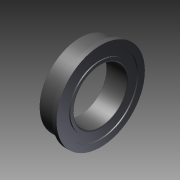
# Autodesk Inventor part: FL6700ZZ
Saved by Autodesk Inventor 2011 SP1 (Build 150282100, 282)
## iProperties
Created: 2017-08-07
Part Number: FL6700ZZ
Catalog Web Link: www.cadenas.de
Description: FL6 _ _ ZZ, FL6 _ _ AZZ, SFL6 _ _ ZZ, SFL6 _ _ AZZ, MFL1 _ _ ZZ, SMFL1 _ _ ZZ-Flanged Ball Bearings (Small Diameter, Deep Groove) - Double Shield Type
Vendor: MISUMI
Document SubType Name: Modeling
Designer: psAdmin
Manufacturer: MISUMI
Mass: 0.398617 g
Surface Area: 6.32309 cm^2
Volume: 0.398617 cm^3
Density: 1 g/cm^3
Category: PARTsolutions
Company: MISUMI
Title: FL6700ZZ
Author: Cadenas PARTsolutions
Comments: Flanged Ball Bearings (Small Diameter, Deep Groove) - Double Shield Type
PSOL_IDENT_0: {$CADENAS_DATA\23d-libs\misumi\metric\12_bearing_holders\sfl608zz.prj},233 {VTYP=3D},{NB=FL6700ZZ},{
PSOL_IDENT_1: LINA=FL6700ZZ},{NN=FL6 _ _ ZZ, FL6 _ _ AZZ, SFL6 _ _ ZZ, SFL6 _ _ AZZ, MFL1 _ _ ZZ, SMFL1 _ _ ZZ},{D
PSOL_IDENT_2: ATE=25.04.2017 02:57:50},{GEOMDATE=28.10.2009 00:00:00},{VERSION=},{LINEID=160},{LINESUBID=-1},{WBVA
PSOL_IDENT_3: R=MAT}  {NB=FL6700ZZ},{LINA=FL6700ZZ},{KT=DUMMY},{PN=FL6700ZZ},{MAT=},{MAT1= '', '52100 Bearing Stee
PSOL_IDENT_4: l', 'S', '440C Stainless Steel'},{BN=6700ZZ},{DD=10.0},{AA=3.6000},{BB=0.5000},{C1=0.7000},{D=15},{B=
PSOL_IDENT_5: 4.0},{D1=16.5},{C=0.8},{RR=0.15},{CR=855},{COR=435},{CRS=855},{CRSS=684},{CORS=435},{CORSS=348},{DS=
PSOL_IDENT_6: 10.30},{R=0.15},{MASS=2.1},{MAT11=1},{MMMM=}
NN: FL6 _ _ ZZ, FL6 _ _ AZZ, SFL6 _ _ ZZ, SFL6 _ _ AZZ, MFL1 _ _ ZZ, SMFL1 _ _ ZZ
NT: Flanged Ball Bearings (Small Diameter, Deep Groove) - Double Shield Type
NB: FL6700ZZ
NBSYN: $PN.
LINA: FL6700ZZ
PN: FL6700ZZ
MAT: 52100 Bearing Steel
BN: 6700ZZ
DD: 10.0
D: 15
B: 4.0
D1: 16.5
C: 0.8
RR: 0.15
CR: 855
COR: 435
DS: 10.30
R: 0.15
MASS: 2.1
SUPPLIER: MISUMI
ARTICLENO: FL6700ZZ
BOMINFO: FL6700ZZ
CREATOR: CADENAS GmbH
Autodesk Inventor part; units mm, degrees
ref_plane "YZ Plane" through (0, 0, 0) normal (1, 0, 0) x (0, 1, 0)
ref_plane "XZ Plane" through (0, 0, 0) normal (0, 1, 0) x (-1, 0, 0)
ref_plane "XY Plane" through (0, 0, 0) normal (0, 0, 1) x (1, 0, 0)
sketch "Sketch_1" plane through (0, 0, 0) normal (0, 0, 1) x (1, 0, 0)
  line L0 (15, 0) -> (-15, 0)
  arc A0 (0, 5.15) -> (0.15, 5) centre (0.15, 5.15) ccw
  line L1 (0.15, 5) -> (3.85, 5)
  arc A1 (3.85, 5) -> (4, 5.15) centre (3.85, 5.15) ccw
  line L2 (4, 5.15) -> (4, 5.7)
  line L3 (4, 5.7) -> (3.8, 5.7)
  line L4 (3.8, 5.7) -> (3.8, 7)
  line L5 (3.8, 7) -> (4, 7)
  line L6 (4, 7) -> (4, 8.25)
  line L7 (4, 8.25) -> (3.2, 8.25)
  line L8 (3.2, 8.25) -> (3.2, 7.65)
  arc A2 (3.05, 7.5) -> (3.2, 7.65) centre (3.2, 7.5) ccw
  line L9 (3.05, 7.5) -> (0.15, 7.5)
  arc A3 (0.15, 7.5) -> (0, 7.35) centre (0.15, 7.35) ccw
  line L10 (0, 7.35) -> (0, 7)
  line L11 (0, 7) -> (0.2, 7)
  line L12 (0.2, 7) -> (0.2, 5.7)
  line L13 (0.2, 5.7) -> (0, 5.7)
  line L14 (0, 5.7) -> (0, 5.15)
  constraints: 30 end point, 8 point on circle, 4 centre point
revolve "Revolution1" add sketch "Sketch_1" angle 360 about axis through (15, 0, 0) along (1, 0, 0)
ref_plane "to_housing_XY" through (0, 0, 0) normal (1, 0, 0) x (0, 0, -1)
ref_plane "to_housing_YZ" through (0, 0, 0) normal (0, 0, -1) x (0, 1, 0)
ref_plane "to_housing_ZX" through (0, 0, 0) normal (0, 1, 0) x (1, 0, 0)
body "Solid1"
